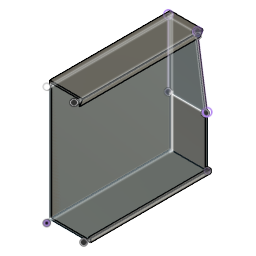
back_cover (Autodesk Fusion 360 design; units mm, degrees)
part number: 2026-08-18-20-48-43-354
Autodesk Fusion 360 part; units mm, degrees
sketch "Sketch1" plane through (0, 0, 0) normal (1, 0, 0) x (0, 1, 0)
  line L0 (0, 0) -> (64.3, 0)
  line L1 (0, 0) -> (1, 0)
  line L2 (64.3, 0) -> (63.3, 0)
  line L3 (64.3, 0) -> (64.3, 60.5)
  line L4 (0, 60.5) -> (64.3, 60.5)
  line L5 (63.3, 0) -> (63.3, 60.5)
  line L6 (1, 0) -> (1, 60.5)
  line L7 (63.3, 59.5) -> (1, 59.5)
  line L8 (1, 1) -> (63.3, 1)
  line L9 (64.3, 0) -> (64.3, 26.12)
  line L10 (64.3, 0) -> (64.3, 26.12)
  line L11 (64.3, 26.12) -> (63.3, 26.12)
  dimension "d1" = 64.3
  dimension "d2" = 1
  dimension "d3" = 1
  dimension "d4" = 60.5
  dimension "d5" = 60.5
  dimension "d6" = 1
  dimension "d7" = 1
  dimension "d19" = 26.12
  constraint coincident L0.start L1.start
  constraint horizontal L0
  constraint parallel L0 L1
  constraint parallel L0 L2
  constraint perpendicular L0 L3
  constraint coincident L4 L5.end
  constraint perpendicular L4 L5
  constraint coincident L4 L6.end
  constraint perpendicular L4 L6
  constraint coincident L5 L7.start
  constraint coincident L6 L7.end
  constraint perpendicular L6 L7
  constraint coincident L6 L8.start
  constraint coincident L5 L8.end
  constraint perpendicular L5 L8
  constraint coincident L3 L9.end
  constraint coincident L5 L11.end
  constraint perpendicular L5 L11
  measures "d1" distance of L0.start L0.end
  measures "d2" distance of L0.start L1.end
  measures "d3" distance of L0.end L2.end
  measures "d4" distance of L0.end L3.end
  measures "d5" distance of L0.start L4.start
  measures "d6" distance of L5.end L7.start
  measures "d7" distance of L1.end L8.start
  measures "d19" distance of L0.end L9.end
extrude "Extrude1" add sketch "Sketch1" against normal blind 1 contours L5 L6 L7 L8 makes body 1
extrude "Extrude2" add sketch "Sketch1" along normal blind 18 separate body contours L0 L5 L6 L8 makes body 2
extrude "Extrude3" add sketch "Sketch1" along normal blind 13 separate body contours L4 L5 L6 L7 makes body 3
extrude "Extrude4" add sketch "Sketch1" against normal blind 1 contours L4 L5 L6 L7 bodies 1 3
extrude "Extrude5" add 1 faces at (-0.6667, 21.7667, 1) along direction (0, 0, -1) blind 1 on bodies 1 bodies 1 2
extrude "Extrude6" add sketch "Sketch1" along normal up to surface (18 mm away) separate body contours L0 L2 L3 L5 L9 L10 L11 makes body 4
extrude "Extrude7" add sketch "Sketch1" against normal blind 1 contours L0 L2 L3 L5 L9 L10 L11 bodies 1 4
sketch "Sketch2" plane through (0, 64.3, 0) normal (0, 1, 0) x (-1, 0, 0)
  line L0 (-18, 26.12) -> (-18, 0)
  line L1 (-18, 0) -> (1, 0)
  line L2 (1, 0) -> (1, 26.12)
  line L3 (1, 26.12) -> (-18, 26.12)
  line L4 (-18, 26.12, -1) -> (-13, 59.5, -1)
  line L5 (1, 60.5, -1) -> (1, 26.12, -1)
  line L6 (-13, 59.5, -1) -> (1, 59.5, -1)
  line L7 (1, 26.12, -1) -> (1, 59.5, -1)
  line L8 (1, 26.12, -1) -> (-18, 26.12, -1)
  point P0 (-18, 26.12)
  point P1 (-13, 59.5)
  constraint coincident P0 L0.start
  constraint coincident L2.end L3.start
extrude "Extrude8" add 1 faces at (-0.6667, 63.3, 48.7067) along direction (0, 1, 0) blind 1 on bodies 1 bodies 1
extrude "Extrude9" cut sketch "Sketch2" along normal blind 1 contours L4 L5 L6 L7 L8 in plane through (0, 63.3, 0) normal (0, 1, 0) bodies 1
extrude "Extrude10" add sketch "Sketch2" along normal blind 1 contours L4 L5 L6 L7 L8 in plane through (0, 63.3, 0) normal (0, 1, 0) bodies 1
sketch "Sketch3" plane through (0, 0, 1) normal (0, 0, 1) x (-1, 0, 0)
  line L0 (0, -63.3) -> (0, -1)
  line L1 (0, -1) -> (-18, -1)
  line L2 (-18, -1) -> (-18, -63.3)
  line L3 (-18, -63.3) -> (0, -63.3)
  line L4 (-18, -1, -1) -> (-18, -64.3, -1)
  line L5 (-18, -64.3, -1) -> (-19, -64.3, -1)
  line L6 (-19, -64.3, -1) -> (-19, -1, -1)
  line L7 (-19, -1, -1) -> (-18, -1, -1)
  line L8 (-13, -64.3, 58.5) -> (-14, -64.3, 58.5)
  line L9 (-13, -1, 58.5) -> (-14, -1, 58.5)
  line L10 (-14, -1, 58.5) -> (-14, -64.3, 58.5)
  line L11 (-13, -64.3, 58.5) -> (-13, -1, 58.5)
  line L12 (-13, -64.3, 58.5) -> (-18, -64.3, 25.12)
  line L13 (-14, -64.3, 58.5) -> (-13.28, -64.3, 56.6305)
  line L14 (-13.28, -64.3, 56.6305) -> (-13, -64.3, 58.5)
  point P0 (-18, -1)
  point P1 (-18, -64.3)
  point P2 (-13, -64.3)
  point P3 (-13, -1)
  dimension "d30" = 1
  dimension "d31" = 1
  dimension "d32" = 1
  constraint coincident P0 L1.end
extrude "Extrude11" add sketch "Sketch3" along normal blind 1 contours L8 L9 L10 L11 in plane through (0, 0, 59.5) normal (0, 0, 1) bodies 1
extrude "Extrude12" add sketch "Sketch3" along normal up to surface (63.3 mm away) contours L8 L12 L13 L14 in plane through (0, 64.3, 1) normal (0, -1, 0) bodies 1
extrude "Extrude13" add sketch "Sketch3" along normal blind 2 contours L4 L5 L6 L7 in plane through (0, 0, 0) normal (0, 0, 1) bodies 1
extrude "Extrude14" add 1 faces at (8.3333, 43.2, 60.5) along direction (0, 0, 1) blind 1 on bodies 1 bodies 1
extrude "Extrude15" cut 1 faces at (8.6667, 21.7667, 59.5) along direction (0, 0, 1) blind 1 on bodies 1 bodies 1
extrude "Extrude16" cut 1 faces at (-0.6667, 1, 20.8333) along direction (0, 1, 0) blind 1 on bodies 1 bodies 1
extrude "Extrude17" cut 1 faces at (-0.6667, 2, 20.8333) along direction (0, 1, 0) blind 0.5 on bodies 1 bodies 1
extrude "Extrude18" add 1 faces at (19, 43.7, 0.6667) along direction (1, 0, 0) blind 1 on bodies 1 bodies 1
extrude "Extrude19" cut 1 faces at (18, 22.7667, 1.3333) along direction (1, 0, 0) blind 1 on bodies 1 bodies 1
extrude "Extrude20" add 1 faces at (14, 23.1, 60.1667) along direction (1, 0, 0) blind 1 on bodies 1 bodies 1
extrude "Extrude21" add 1 faces at (13.76, 43.3667, 58.8768) along direction (0.933195, 0, -0.359372) blind 1 on bodies 1 bodies 1
extrude "Extrude22" cut 1 faces at (13.0933, 43.0333, 58.8768) along direction (0.988967, 0, 0.148138) blind 1 on bodies 1 bodies 1
extrude "Extrude23" cut 1 faces at (13, 43.0333, 60.1667) along direction (1, 0, 0) blind 1 on bodies 1 bodies 1
extrude "Extrude24" cut 1 faces at (13.9394, 22.7667, 57.7292) along direction (0.148138, 0, -0.988967) blind 1 on bodies 1 bodies 1
extrude "Extrude25" add 1 faces at (14.6261, 43.3667, 59.2589) along direction (0.359372, 0, 0.933195) up to surface end surface through (14, 2.5, 61.5) normal (0, 0, 1) offset 0 on bodies 1 bodies 1
extrude "Extrude26" cut 1 faces at (13.9022, 63.6333, 57.3909) along direction (0.359372, 0, 0.933195) blind 0.264 on bodies 1 bodies 1
extrude "Extrude27" add 1 faces at (3.6667, 43.7, 61.5) along direction (0, 0, 1) blind 0.25 on bodies 1 bodies 1
extrude "Extrude28" cut 1 faces at (9, 43.0333, 60.5) along direction (0, 0, 1) blind 0.25 on bodies 1 bodies 1
